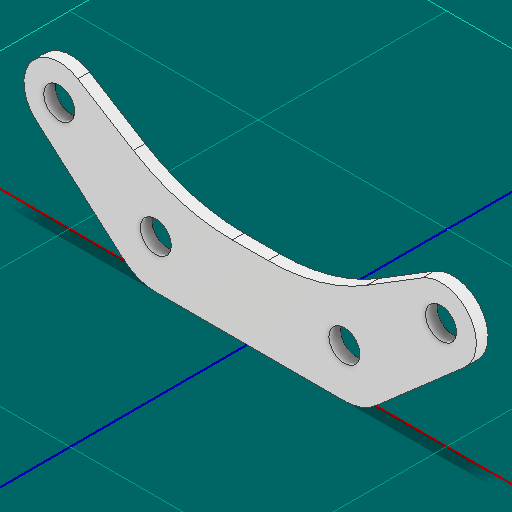
# Autodesk Inventor part: Hook Gusset Brace
Saved by Autodesk Inventor 2025 (Build 290162000, 162)
## iProperties
Created: 2024-10-13
Part Number: Hook Gusset Brace
Material: Acetal Resin, White
Document SubType Name: Modeling
Designer: Averey Ku
Density: 1.425 g/cm^3
Appearance: Smooth - White
Author: Averey Ku
Autodesk Inventor part; units mm, degrees
ref_plane "YZ Plane" through (0, 0, 0) normal (1, 0, 0) x (0, 1, 0)
ref_plane "XZ Plane" through (0, 0, 0) normal (0, 1, 0) x (-1, 0, 0)
ref_plane "XY Plane" through (0, 0, 0) normal (0, 0, 1) x (1, 0, 0)
sketch "Sketch1" plane through (0, 0, 0) normal (0, 0, 1) x (1, 0, 0)
  circle A0 centre (13.2036, 20.3187) radius 2.0955
  circle A1 centre (-12.1964, 20.3187) radius 2.0955
  line L0 (2.9057, 25.0812) -> (-1.8984, 25.0812)
  circle A2 centre (-25.2051, 29.4175) radius 2.0955
  arc A3 (-22.7052, 33.4711) -> (-28.3391, 25.8315) centre (-25.2051, 29.4175) ccw
  arc A4 (29.3464, 25.8315) -> (23.7125, 33.4711) centre (26.2124, 29.4175) ccw
  circle A5 centre (26.2124, 29.4175) radius 2.0955
  line L1 (-22.7052, 33.4711) -> (-15.2312, 28.8619)
  line L2 (23.7125, 33.4711) -> (16.2385, 28.8619)
  arc A6 (-15.2312, 28.8619) -> (-1.8984, 25.0812) centre (-1.8984, 50.4812) ccw
  arc A7 (2.9057, 25.0812) -> (16.2385, 28.8619) centre (2.9057, 50.4812) ccw
  arc A8 (-16.4554, 15.4455) -> (-12.1964, 13.8467) centre (-12.1964, 20.3187) ccw
  arc A9 (13.2036, 13.8467) -> (17.4626, 15.4455) centre (13.2036, 20.3187) ccw
  line L3 (-12.1964, 13.8467) -> (13.2036, 13.8467)
  line L4 (-28.3391, 25.8315) -> (-16.4554, 15.4455)
  line L5 (17.4626, 15.4455) -> (29.3464, 25.8315)
  circle A10 centre (-12.1964, 20.3187) radius 3.6662
  circle A11 centre (13.2036, 20.3187) radius 3.6662
  point P0 (0, 0)
  point P1 (-12.1964, 25.0812)
  point P2 (17.4758, 18.214)
  point P3 (-16.4686, 18.214)
  point P4 (0.5036, 25.0812)
  dimension "d8" = 4.191
  dimension "d9" = 4.191
  dimension "d13" = 4.191
  dimension "d14" = 9.525
  dimension "d15" = 9.525
  dimension "d16" = 4.191
  dimension "d17" = 25.4
  dimension "d19" = 7.3323
  dimension "d21" = 15.875
  dimension "d23" = 15.875
  constraints: 13 tangent, 12 centre point, 12 end point, 12 point on circle, 6 coincident, 2 horizontal, 1 equal radius, 1 midpoint, 4 other
  measures "d8" diameter of A1
  measures "d9" diameter of A0
  measures "d13" diameter of A2
  measures "d14" diameter of A3
  measures "d15" diameter of A4
  measures "d16" diameter of A5
  measures "d17" radius of A6
  measures "d19" diameter of A10
  measures "d21" distance of A1.centre A2.centre
  measures "d23" distance of A4.centre A0.centre
extrude "Extrusion1" add sketch "Sketch1" along normal blind 1.5875 contours A7 L2 A4 L5 A9 L3 A8 L4 A3 L1 A6 L0 | A10 | A11
body "Solid1"
